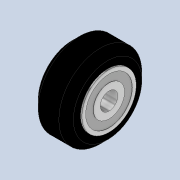
# Autodesk Inventor part: M5 V Wheel
Saved by Autodesk Inventor 2022 (Build 260153000, 153)
## iProperties
Created: 2021-10-14
Part Number: M5 V Wheel
Material: Generic
Document SubType Name: Modeling
Designer: Coy
Density: 1 g/cm^3
Appearance: Chrome - Polished
Author: Coy
Autodesk Inventor part; units mm, degrees
ref_plane "YZ Plane" through (0, 0, 0) normal (1, 0, 0) x (0, 1, 0)
ref_plane "XZ Plane" through (0, 0, 0) normal (0, 1, 0) x (-1, 0, 0)
sketch "Sketch1" plane through (0, 0, 0) normal (1, 0, 0) x (0, 1, 0)
  circle A0 centre (0, 0) radius 2.525
  circle A1 centre (0, 0) radius 7.85
  dimension "d0" = 5.05
  dimension "d1" = 15.7
  constraints: 2 centre point, 2 coincident
  measures "d0" diameter of A0
  measures "d1" diameter of A1
extrude "Extrusion1" add sketch "Sketch1" against normal blind 11
sketch "Sketch2" plane through (0, 0, 0) normal (1, 0, 0) x (0, 0, -1)
  circle A0 centre (0, 0) radius 4.5
  circle A1 centre (0, 0) radius 6.75
  dimension "d4" = 9
  dimension "d5" = 13.5
  constraints: 2 centre point, 2 coincident
  measures "d4" diameter of A0
  measures "d5" diameter of A1
extrude "Extrusion2" cut sketch "Sketch2" against normal blind 0.1
sketch "Sketch3" plane through (-11, 0, 0) normal (-1, 0, 0) x (0, 0, 1)
  circle A0 centre (0, 0) radius 6.75 projected
  circle A1 centre (0, 0) radius 4.5 projected
extrude "Extrusion3" cut sketch "Sketch3" against normal blind 0.1
ref_plane "Work Plane1" through (-0.4, 0, 0) normal (1, 0, 0) x (0, 0, -1)
sketch "Sketch4" plane through (-0.4, 0, 0) normal (1, 0, 0) x (0, 0, -1)
  circle A0 centre (0, 0) radius 7.85 projected
  circle A1 centre (0, 0) radius 12
  dimension "d11" = 24
  constraints: 1 centre point, 1 coincident
  measures "d11" diameter of A1
extrude "Extrusion4" add sketch "Sketch4" against normal blind 10.2
chamfer "Chamfer1" distance 2.1 angle 45 1 edges at (-0.4, 0, 12) measured on face at (-0.4, -1.2727, -10.4814)
chamfer "Chamfer2" distance 2.1 angle 45 1 edges at (-10.6, 0, 12) measured on face at (-10.6, -1.2727, -10.4814)
body "Solid1"
